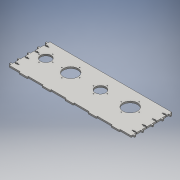
# Autodesk Inventor part: PLANO  N°1
Saved by Autodesk Inventor 2016 (Build 200138000, 138)
## iProperties
Created: 2017-09-26
Part Number: PLANO  N°1
Material: Genérico
Document SubType Name: Modeling
Designer: Alumno
Density: 1 g/cm^3
Appearance: Valor por defecto
Author: Alumno
Autodesk Inventor part; units mm, degrees
ref_plane "YZ Plane" through (0, 0, 0) normal (1, 0, 0) x (0, 1, 0)
ref_plane "XZ Plane" through (0, 0, 0) normal (0, 1, 0) x (-1, 0, 0)
ref_plane "XY Plane" through (0, 0, 0) normal (0, 0, 1) x (1, 0, 0)
sketch "Boceto1" plane through (0, 0, 0) normal (0, 0, 1) x (1, 0, 0)
  circle A0 centre (-88.2, 15) radius 27
  circle A1 centre (131.4, 15) radius 27
  circle A2 centre (21.6, 15) radius 19.5
  circle A3 centre (-180, 15) radius 19.5
  line L0 (225, 16.7667) -> (218.8, 16.7667)
  line L1 (218.8, 16.7667) -> (218.8, 15.4667)
  line L2 (218.8, 15.4667) -> (216, 15.4667)
  line L3 (216, 15.4667) -> (216, 16.7667)
  line L4 (216, 16.7667) -> (210, 16.7667)
  line L5 (210, 16.7667) -> (210, 20.1167)
  line L6 (210, 20.1167) -> (216, 20.1167)
  line L7 (216, 20.1167) -> (216, 21.4167)
  line L8 (216, 21.4167) -> (218.8, 21.4167)
  line L9 (218.8, 21.4167) -> (218.8, 20.1167)
  line L10 (218.8, 20.1167) -> (225, 20.1167)
  line L11 (225, 20.1167) -> (225, 34.3833)
  line L12 (225, 39.3833) -> (225, 53.65)
  line L13 (225, 53.65) -> (218.8, 53.65)
  line L14 (218.8, 53.65) -> (218.8, 52.35)
  line L15 (218.8, 52.35) -> (216, 52.35)
  line L16 (216, 52.35) -> (216, 53.65)
  line L17 (216, 53.65) -> (210, 53.65)
  line L18 (210, 53.65) -> (210, 57)
  line L19 (210, 57) -> (216, 57)
  line L20 (216, 57) -> (216, 58.3)
  line L21 (216, 58.3) -> (218.8, 58.3)
  line L22 (218.8, 58.3) -> (218.8, 57)
  line L23 (218.8, 57) -> (225, 57)
  line L24 (225, 57) -> (225, 63.9297)
  line L25 (225, 63.9297) -> (231, 63.9297)
  line L26 (231, 68.9297) -> (231, 63.9297)
  line L27 (225, 68.9297) -> (231, 68.9297)
  line L28 (225, 68.9297) -> (225, 75)
  line L29 (225, 75) -> (-225, 75)
  line L30 (-225, 75) -> (-225, 68.9297)
  line L31 (-225, 68.9297) -> (-231, 68.9297)
  line L32 (-231, 68.9297) -> (-231, 63.9297)
  line L33 (-231, 63.9297) -> (-225, 63.9297)
  line L34 (-225, 63.9297) -> (-225, 57)
  line L35 (-225, 57) -> (-218.8, 57)
  line L36 (-218.8, 57) -> (-218.8, 58.3)
  line L37 (-218.8, 58.3) -> (-216, 58.3)
  line L38 (-216, 58.3) -> (-216, 57)
  line L39 (-216, 57) -> (-210, 57)
  line L40 (-210, 57) -> (-210, 53.65)
  line L41 (-210, 53.65) -> (-216, 53.65)
  line L42 (-216, 53.65) -> (-216, 52.35)
  line L43 (-216, 52.35) -> (-218.8, 52.35)
  line L44 (-218.8, 52.35) -> (-218.8, 53.65)
  line L45 (-218.8, 53.65) -> (-225, 53.65)
  line L46 (-225, 53.65) -> (-225, 39.3833)
  line L47 (-225, 39.3833) -> (-231, 39.3833)
  line L48 (-231, 39.3833) -> (-231, 34.3833)
  line L49 (-231, 34.3833) -> (-225, 34.3833)
  line L50 (-225, 34.3833) -> (-225, 20.1167)
  line L51 (-225, 20.1167) -> (-218.8, 20.1167)
  line L52 (-218.8, 20.1167) -> (-218.8, 21.4167)
  line L53 (-218.8, 21.4167) -> (-216, 21.4167)
  line L54 (-216, 21.4167) -> (-216, 20.1167)
  line L55 (-216, 20.1167) -> (-210, 20.1167)
  line L56 (-210, 20.1167) -> (-210, 16.7667)
  line L57 (-210, 16.7667) -> (-216, 16.7667)
  line L58 (-216, 16.7667) -> (-216, 15.4667)
  line L59 (-216, 15.4667) -> (-218.8, 15.4667)
  line L60 (-218.8, 15.4667) -> (-218.8, 16.7667)
  line L61 (-218.8, 16.7667) -> (-225, 16.7667)
  line L62 (-225, 16.7667) -> (-225, 2.5)
  line L63 (-225, 2.5) -> (-231, 2.5)
  line L64 (-231, 2.5) -> (-231, -2.5)
  line L65 (-231, -2.5) -> (-225, -2.5)
  line L66 (-225, -2.5) -> (-225, -16.7667)
  line L67 (-225, -16.7667) -> (-218.8, -16.7667)
  line L68 (-218.8, -16.7667) -> (-218.8, -15.4667)
  line L69 (-218.8, -15.4667) -> (-216, -15.4667)
  line L70 (-216, -15.4667) -> (-216, -16.7667)
  line L71 (-216, -16.7667) -> (-210, -16.7667)
  line L72 (-210, -16.7667) -> (-210, -20.1167)
  line L73 (-210, -20.1167) -> (-216, -20.1167)
  line L74 (-216, -20.1167) -> (-216, -21.4167)
  line L75 (-216, -21.4167) -> (-218.8, -21.4167)
  line L76 (-218.8, -21.4167) -> (-218.8, -20.1167)
  line L77 (-218.8, -20.1167) -> (-225, -20.1167)
  line L78 (-225, -20.1167) -> (-225, -34.3833)
  line L79 (-225, -34.3833) -> (-231, -34.3833)
  line L80 (-231, -34.3833) -> (-231, -39.3833)
  line L81 (-231, -39.3833) -> (-225, -39.3833)
  line L82 (-225, -39.3833) -> (-225, -53.65)
  line L83 (-225, -53.65) -> (-218.8, -53.65)
  line L84 (-218.8, -53.65) -> (-218.8, -52.35)
  line L85 (-218.8, -52.35) -> (-216, -52.35)
  line L86 (-216, -52.35) -> (-216, -53.65)
  line L87 (-216, -53.65) -> (-210, -53.65)
  line L88 (-210, -53.65) -> (-210, -57)
  line L89 (-210, -57) -> (-216, -57)
  line L90 (-216, -57) -> (-216, -58.3)
  line L91 (-216, -58.3) -> (-218.8, -58.3)
  line L92 (-218.8, -58.3) -> (-218.8, -57)
  line L93 (-218.8, -57) -> (-225, -57)
  line L94 (-225, -57) -> (-225, -63.5)
  line L95 (-225, -63.5) -> (-231, -63.5)
  line L96 (-231, -63.5) -> (-231, -68.5)
  line L97 (-231, -68.5) -> (-225, -68.5)
  line L98 (-225, -68.5) -> (-225, -75)
  line L99 (-225, -75) -> (-185, -75)
  line L100 (-185, -75) -> (-185, -79)
  line L101 (-185, -79) -> (-155, -79)
  line L102 (-155, -79) -> (-155, -75)
  line L103 (-155, -75) -> (-100, -75)
  line L104 (-100, -75) -> (-100, -79)
  line L105 (-100, -79) -> (-70, -79)
  line L106 (-70, -79) -> (-70, -75)
  line L107 (-70, -75) -> (-15, -75)
  line L108 (-15, -75) -> (-15, -79)
  line L109 (-15, -79) -> (15, -79)
  line L110 (15, -79) -> (15, -75)
  line L111 (15, -75) -> (70, -75)
  line L112 (70, -75) -> (70, -79)
  line L113 (70, -79) -> (100, -79)
  line L114 (100, -79) -> (100, -75)
  line L115 (100, -75) -> (155, -75)
  line L116 (155, -79) -> (155, -75)
  line L117 (185, -79) -> (155, -79)
  line L118 (185, -75) -> (185, -79)
  line L119 (185, -75) -> (225, -75)
  line L120 (225, -75) -> (225, -68.5)
  line L121 (225, -68.5) -> (231, -68.5)
  line L122 (231, -63.5) -> (231, -68.5)
  line L123 (225, -63.5) -> (231, -63.5)
  line L124 (225, -63.5) -> (225, -57)
  line L125 (225, -57) -> (218.8, -57)
  line L126 (218.8, -57) -> (218.8, -58.3)
  line L127 (218.8, -58.3) -> (216, -58.3)
  line L128 (216, -58.3) -> (216, -57)
  line L129 (216, -57) -> (210, -57)
  line L130 (210, -57) -> (210, -53.65)
  line L131 (210, -53.65) -> (216, -53.65)
  line L132 (216, -53.65) -> (216, -52.35)
  line L133 (216, -52.35) -> (218.8, -52.35)
  line L134 (218.8, -52.35) -> (218.8, -53.65)
  line L135 (218.8, -53.65) -> (225, -53.65)
  line L136 (225, -53.65) -> (225, -39.3833)
  line L137 (225, -39.3833) -> (231, -39.3833)
  line L138 (231, -34.3833) -> (231, -39.3833)
  line L139 (225, -34.3833) -> (231, -34.3833)
  line L140 (225, -34.3833) -> (225, -20.1167)
  line L141 (225, -20.1167) -> (218.8, -20.1167)
  line L142 (218.8, -20.1167) -> (218.8, -21.4167)
  line L143 (218.8, -21.4167) -> (216, -21.4167)
  line L144 (216, -21.4167) -> (216, -20.1167)
  line L145 (216, -20.1167) -> (210, -20.1167)
  line L146 (210, -20.1167) -> (210, -16.7667)
  line L147 (210, -16.7667) -> (216, -16.7667)
  line L148 (216, -16.7667) -> (216, -15.4667)
  line L149 (216, -15.4667) -> (218.8, -15.4667)
  line L150 (218.8, -15.4667) -> (218.8, -16.7667)
  line L151 (218.8, -16.7667) -> (225, -16.7667)
  line L152 (225, -16.7667) -> (225, -2.5)
  line L153 (225, -2.5) -> (231, -2.5)
  line L154 (231, 2.5) -> (231, -2.5)
  line L155 (225, 2.5) -> (231, 2.5)
  line L156 (225, 2.5) -> (225, 16.7667)
  line L157 (225, 39.3833) -> (231, 39.3833)
  line L158 (231, 39.3833) -> (231, 34.3833)
  line L159 (231, 34.3833) -> (225, 34.3833)
  point P0 (0, 0)
  point P1 (0, 0)
  dimension "d0" = 450
  dimension "d1" = 150
  dimension "d6" = 54
  dimension "d7" = 60
  dimension "d9" = 90
  dimension "d10" = 45
  dimension "d11" = 91.8
  dimension "d12" = 39
  dimension "d14" = 90
  dimension "d15" = 39
  dimension "d16" = 90
  dimension "d17" = 14.2667
  dimension "d19" = 54
  dimension "d20" = 109.8
  dimension "d21" = 109.8
  dimension "d58" = 6.2
  dimension "d59" = 6.2
  dimension "d60" = 2.8
  dimension "d61" = 2.8
  dimension "d62" = 450
  dimension "d63" = 450
  dimension "d64" = 450
  dimension "d65" = 450
  dimension "d67" = 15
  dimension "d68" = 15
  dimension "d69" = 6
  dimension "d70" = 5
  constraints: 320 end point, 4 centre point, 2 perpendicular, 1 horizontal
  measures "d0" distance of L29.start L29.end
  measures "d1" distance between parallel lines of L103 L29
  measures "d6" diameter of A0
  measures "d7" distance from line of L29 A0.centre
  measures "d9" distance from line of L99 A3.centre
  measures "d10" distance from line of A3.centre L50
  measures "d11" distance of A0.centre A3.centre
  measures "d12" diameter of A3
  measures "d14" distance from line of L107 A2.centre
  measures "d15" diameter of A2
  measures "d16" distance from line of L115 A1.centre
  measures "d17" distance of L10.end L11.end
  measures "d19" diameter of A1
  measures "d20" distance of A2.centre A0.centre
  measures "d21" distance of A1.centre A2.centre
  measures "d58" distance of L22.end L23.end
  measures "d59" distance of L13.start L14.start
  measures "d60" distance of L15.start L16.start
  measures "d61" distance of L20.end L22.start
  measures "d62" distance from line of L120 L98.end
  measures "d63" distance between parallel lines of L30 L12
  measures "d64" distance between parallel lines of L30 L11
  measures "d65" distance between parallel lines of L30 L156
  measures "d67" distance between parallel lines of L24 L18
  measures "d68" distance between parallel lines of L11 L5
  measures "d69" distance of L12.start L157.end
  measures "d70" distance of L157.end L158.end
extrude "Extrusión1" add sketch "Boceto1" along normal blind 6
sketch "Boceto2" plane through (0, 0, 6) normal (0, 0, 1) x (1, 0, 0)
  circle A0 centre (-88.2, 15) radius 27 projected
  circle A1 centre (131.4, 15) radius 27 projected
  circle A2 centre (-180, 15) radius 19.5 projected
  circle A3 centre (21.6, 15) radius 19.5 projected
  line L0 (225, 16.7667) -> (218.8, 16.7667) projected
  line L1 (218.8, 16.7667) -> (218.8, 15.4667) projected
  line L2 (218.8, 15.4667) -> (216, 15.4667) projected
  line L3 (216, 15.4667) -> (216, 16.7667) projected
  line L4 (216, 16.7667) -> (210, 16.7667) projected
  line L5 (210, 16.7667) -> (210, 20.1167) projected
  line L6 (210, 20.1167) -> (216, 20.1167) projected
  line L7 (216, 20.1167) -> (216, 21.4167) projected
  line L8 (216, 21.4167) -> (218.8, 21.4167) projected
  line L9 (218.8, 21.4167) -> (218.8, 20.1167) projected
  line L10 (218.8, 20.1167) -> (225, 20.1167) projected
  line L11 (225, 20.1167) -> (225, 34.3833) projected
  line L12 (225, 39.3833) -> (225, 53.65) projected
  line L13 (225, 53.65) -> (218.8, 53.65) projected
  line L14 (218.8, 53.65) -> (218.8, 52.35) projected
  line L15 (218.8, 52.35) -> (216, 52.35) projected
  line L16 (216, 52.35) -> (216, 53.65) projected
  line L17 (216, 53.65) -> (210, 53.65) projected
  line L18 (210, 53.65) -> (210, 57) projected
  line L19 (210, 57) -> (216, 57) projected
  line L20 (216, 57) -> (216, 58.3) projected
  line L21 (216, 58.3) -> (218.8, 58.3) projected
  line L22 (218.8, 58.3) -> (218.8, 57) projected
  line L23 (218.8, 57) -> (225, 57) projected
  line L24 (225, 57) -> (225, 63.9297) projected
  line L25 (225, 63.9297) -> (231, 63.9297) projected
  line L26 (231, 63.9297) -> (231, 68.9297) projected
  line L27 (231, 68.9297) -> (225, 68.9297) projected
  line L28 (225, 68.9297) -> (225, 75) projected
  line L29 (225, 75) -> (-225, 75) projected
  line L30 (-225, 75) -> (-225, 68.9297) projected
  line L31 (-225, 68.9297) -> (-231, 68.9297) projected
  line L32 (-231, 68.9297) -> (-231, 63.9297) projected
  line L33 (-231, 63.9297) -> (-225, 63.9297) projected
  line L34 (-225, 63.9297) -> (-225, 57) projected
  line L35 (-225, 57) -> (-218.8, 57) projected
  line L36 (-218.8, 57) -> (-218.8, 58.3) projected
  line L37 (-218.8, 58.3) -> (-216, 58.3) projected
  line L38 (-216, 58.3) -> (-216, 57) projected
  line L39 (-216, 57) -> (-210, 57) projected
  line L40 (-210, 57) -> (-210, 53.65) projected
  line L41 (-210, 53.65) -> (-216, 53.65) projected
  line L42 (-216, 53.65) -> (-216, 52.35) projected
  line L43 (-216, 52.35) -> (-218.8, 52.35) projected
  line L44 (-218.8, 52.35) -> (-218.8, 53.65) projected
  line L45 (-218.8, 53.65) -> (-225, 53.65) projected
  line L46 (-225, 53.65) -> (-225, 39.3833) projected
  line L47 (-225, 39.3833) -> (-231, 39.3833) projected
  line L48 (-231, 39.3833) -> (-231, 34.3833) projected
  line L49 (-231, 34.3833) -> (-225, 34.3833) projected
  line L50 (-225, 34.3833) -> (-225, 20.1167) projected
  line L51 (-225, 20.1167) -> (-218.8, 20.1167) projected
  line L52 (-218.8, 20.1167) -> (-218.8, 21.4167) projected
  line L53 (-218.8, 21.4167) -> (-216, 21.4167) projected
  line L54 (-216, 21.4167) -> (-216, 20.1167) projected
  line L55 (-216, 20.1167) -> (-210, 20.1167) projected
  line L56 (-210, 20.1167) -> (-210, 16.7667) projected
  line L57 (-210, 16.7667) -> (-216, 16.7667) projected
  line L58 (-216, 16.7667) -> (-216, 15.4667) projected
  line L59 (-216, 15.4667) -> (-218.8, 15.4667) projected
  line L60 (-218.8, 15.4667) -> (-218.8, 16.7667) projected
  line L61 (-218.8, 16.7667) -> (-225, 16.7667) projected
  line L62 (-225, 16.7667) -> (-225, 2.5) projected
  line L63 (-225, 2.5) -> (-231, 2.5) projected
  line L64 (-231, 2.5) -> (-231, -2.5) projected
  line L65 (-231, -2.5) -> (-225, -2.5) projected
  line L66 (-225, -2.5) -> (-225, -16.7667) projected
  line L67 (-225, -16.7667) -> (-218.8, -16.7667) projected
  line L68 (-218.8, -16.7667) -> (-218.8, -15.4667) projected
  line L69 (-218.8, -15.4667) -> (-216, -15.4667) projected
  line L70 (-216, -15.4667) -> (-216, -16.7667) projected
  line L71 (-216, -16.7667) -> (-210, -16.7667) projected
  line L72 (-210, -16.7667) -> (-210, -20.1167) projected
  line L73 (-210, -20.1167) -> (-216, -20.1167) projected
  line L74 (-216, -20.1167) -> (-216, -21.4167) projected
  line L75 (-216, -21.4167) -> (-218.8, -21.4167) projected
  line L76 (-218.8, -21.4167) -> (-218.8, -20.1167) projected
  line L77 (-218.8, -20.1167) -> (-225, -20.1167) projected
  line L78 (-225, -20.1167) -> (-225, -34.3833) projected
  line L79 (-225, -34.3833) -> (-231, -34.3833) projected
  line L80 (-231, -34.3833) -> (-231, -39.3833) projected
  line L81 (-231, -39.3833) -> (-225, -39.3833) projected
  line L82 (-225, -39.3833) -> (-225, -53.65) projected
  line L83 (-225, -53.65) -> (-218.8, -53.65) projected
  line L84 (-218.8, -53.65) -> (-218.8, -52.35) projected
  line L85 (-218.8, -52.35) -> (-216, -52.35) projected
  line L86 (-216, -52.35) -> (-216, -53.65) projected
  line L87 (-216, -53.65) -> (-210, -53.65) projected
  line L88 (-210, -53.65) -> (-210, -57) projected
  line L89 (-210, -57) -> (-216, -57) projected
  line L90 (-216, -57) -> (-216, -58.3) projected
  line L91 (-216, -58.3) -> (-218.8, -58.3) projected
  line L92 (-218.8, -58.3) -> (-218.8, -57) projected
  line L93 (-218.8, -57) -> (-225, -57) projected
  line L94 (-225, -57) -> (-225, -63.5) projected
  line L95 (-225, -63.5) -> (-231, -63.5) projected
  line L96 (-231, -63.5) -> (-231, -68.5) projected
  line L97 (-231, -68.5) -> (-225, -68.5) projected
  line L98 (-225, -68.5) -> (-225, -75) projected
  line L99 (-225, -75) -> (-185, -75) projected
  line L100 (-185, -75) -> (-185, -79) projected
  line L101 (-185, -79) -> (-155, -79) projected
  line L102 (-155, -79) -> (-155, -75) projected
  line L103 (-155, -75) -> (-100, -75) projected
  line L104 (-100, -75) -> (-100, -79) projected
  line L105 (-100, -79) -> (-70, -79) projected
  line L106 (-70, -79) -> (-70, -75) projected
  line L107 (-70, -75) -> (-15, -75) projected
  line L108 (-15, -75) -> (-15, -79) projected
  line L109 (-15, -79) -> (15, -79) projected
  line L110 (15, -79) -> (15, -75) projected
  line L111 (15, -75) -> (70, -75) projected
  line L112 (70, -75) -> (70, -79) projected
  line L113 (70, -79) -> (100, -79) projected
  line L114 (100, -79) -> (100, -75) projected
  line L115 (100, -75) -> (155, -75) projected
  line L116 (155, -75) -> (155, -79) projected
  line L117 (155, -79) -> (185, -79) projected
  line L118 (185, -79) -> (185, -75) projected
  line L119 (185, -75) -> (225, -75) projected
  line L120 (225, -75) -> (225, -68.5) projected
  line L121 (225, -68.5) -> (231, -68.5) projected
  line L122 (231, -68.5) -> (231, -63.5) projected
  line L123 (231, -63.5) -> (225, -63.5) projected
  line L124 (225, -63.5) -> (225, -57) projected
  line L125 (225, -57) -> (218.8, -57) projected
  line L126 (218.8, -57) -> (218.8, -58.3) projected
  line L127 (218.8, -58.3) -> (216, -58.3) projected
  line L128 (216, -58.3) -> (216, -57) projected
  line L129 (216, -57) -> (210, -57) projected
  line L130 (210, -57) -> (210, -53.65) projected
  line L131 (210, -53.65) -> (216, -53.65) projected
  line L132 (216, -53.65) -> (216, -52.35) projected
  line L133 (216, -52.35) -> (218.8, -52.35) projected
  line L134 (218.8, -52.35) -> (218.8, -53.65) projected
  line L135 (218.8, -53.65) -> (225, -53.65) projected
  line L136 (225, -53.65) -> (225, -39.3833) projected
  line L137 (225, -39.3833) -> (231, -39.3833) projected
  line L138 (231, -39.3833) -> (231, -34.3833) projected
  line L139 (231, -34.3833) -> (225, -34.3833) projected
  line L140 (225, -34.3833) -> (225, -20.1167) projected
  line L141 (225, -20.1167) -> (218.8, -20.1167) projected
  line L142 (218.8, -20.1167) -> (218.8, -21.4167) projected
  line L143 (218.8, -21.4167) -> (216, -21.4167) projected
  line L144 (216, -21.4167) -> (216, -20.1167) projected
  line L145 (216, -20.1167) -> (210, -20.1167) projected
  line L146 (210, -20.1167) -> (210, -16.7667) projected
  line L147 (210, -16.7667) -> (216, -16.7667) projected
  line L148 (216, -16.7667) -> (216, -15.4667) projected
  line L149 (216, -15.4667) -> (218.8, -15.4667) projected
  line L150 (218.8, -15.4667) -> (218.8, -16.7667) projected
  line L151 (218.8, -16.7667) -> (225, -16.7667) projected
  line L152 (225, -16.7667) -> (225, -2.5) projected
  line L153 (225, -2.5) -> (231, -2.5) projected
  line L154 (231, -2.5) -> (231, 2.5) projected
  line L155 (231, 2.5) -> (225, 2.5) projected
  line L156 (225, 2.5) -> (225, 16.7667) projected
  circle A4 centre (-88.2, 48) radius 1.5
  circle A5 centre (-121.2, 15) radius 1.5
  circle A6 centre (-88.2, -18) radius 1.5
  circle A7 centre (-55.2, 15) radius 1.5
  circle A8 centre (131.4, 48) radius 1.5
  circle A9 centre (98.4, 15) radius 1.5
  circle A10 centre (131.4, -18) radius 1.5
  circle A11 centre (164.4, 15) radius 1.5
  line L157 (225, 34.3833) -> (231, 34.3833) projected
  line L158 (231, 34.3833) -> (231, 39.3833) projected
  line L159 (231, 39.3833) -> (225, 39.3833) projected
  point P0 (0, 0)
  dimension "d25" = 3
  dimension "d26" = 33
  dimension "d29" = 360
  dimension "d31" = 3
  dimension "d32" = 33
  dimension "d35" = 360
  constraints: 8 centre point, 18 other
  measures "d25" diameter of A4
  measures "d26" distance of A0.centre A4.centre
  measures "d31" diameter of A8
  measures "d32" distance of A1.centre A8.centre
extrude "Extrusión2" cut sketch "Boceto2" against normal blind 6 contours A4 | A5 | A6 | A7 | A8 | A9 | A10 | A11
sketch "Boceto3" plane through (0, 0, 6) normal (0, 0, 1) x (1, 0, 0)
  circle A0 centre (131.4, -18) radius 1.5 projected
  circle A1 centre (131.4, 48) radius 1.5 projected
  circle A2 centre (-88.2, -18) radius 1.5 projected
  circle A3 centre (-88.2, 48) radius 1.5 projected
  circle A4 centre (-121.2, 15) radius 1.5 projected
  circle A5 centre (-55.2, 15) radius 1.5 projected
  circle A6 centre (98.4, 15) radius 1.5 projected
  circle A7 centre (164.4, 15) radius 1.5 projected
  circle A8 centre (-88.2, 15) radius 27 projected
  circle A9 centre (131.4, 15) radius 27 projected
  circle A10 centre (-180, 15) radius 19.5 projected
  circle A11 centre (21.6, 15) radius 19.5 projected
  line L0 (225, 16.7667) -> (218.8, 16.7667) projected
  line L1 (218.8, 16.7667) -> (218.8, 15.4667) projected
  line L2 (218.8, 15.4667) -> (216, 15.4667) projected
  line L3 (216, 15.4667) -> (216, 16.7667) projected
  line L4 (216, 16.7667) -> (210, 16.7667) projected
  line L5 (210, 16.7667) -> (210, 20.1167) projected
  line L6 (210, 20.1167) -> (216, 20.1167) projected
  line L7 (216, 20.1167) -> (216, 21.4167) projected
  line L8 (216, 21.4167) -> (218.8, 21.4167) projected
  line L9 (218.8, 21.4167) -> (218.8, 20.1167) projected
  line L10 (218.8, 20.1167) -> (225, 20.1167) projected
  line L11 (225, 20.1167) -> (225, 34.3833) projected
  line L12 (225, 39.3833) -> (225, 53.65) projected
  line L13 (225, 53.65) -> (218.8, 53.65) projected
  line L14 (218.8, 53.65) -> (218.8, 52.35) projected
  line L15 (218.8, 52.35) -> (216, 52.35) projected
  line L16 (216, 52.35) -> (216, 53.65) projected
  line L17 (216, 53.65) -> (210, 53.65) projected
  line L18 (210, 53.65) -> (210, 57) projected
  line L19 (210, 57) -> (216, 57) projected
  line L20 (216, 57) -> (216, 58.3) projected
  line L21 (216, 58.3) -> (218.8, 58.3) projected
  line L22 (218.8, 58.3) -> (218.8, 57) projected
  line L23 (218.8, 57) -> (225, 57) projected
  line L24 (225, 57) -> (225, 63.9297) projected
  line L25 (225, 63.9297) -> (231, 63.9297) projected
  line L26 (231, 63.9297) -> (231, 68.9297) projected
  line L27 (231, 68.9297) -> (225, 68.9297) projected
  line L28 (225, 68.9297) -> (225, 75) projected
  line L29 (225, 75) -> (-225, 75) projected
  line L30 (-225, 75) -> (-225, 68.9297) projected
  line L31 (-225, 68.9297) -> (-231, 68.9297) projected
  line L32 (-231, 68.9297) -> (-231, 63.9297) projected
  line L33 (-231, 63.9297) -> (-225, 63.9297) projected
  line L34 (-225, 63.9297) -> (-225, 57) projected
  line L35 (-225, 57) -> (-218.8, 57) projected
  line L36 (-218.8, 57) -> (-218.8, 58.3) projected
  line L37 (-218.8, 58.3) -> (-216, 58.3) projected
  line L38 (-216, 58.3) -> (-216, 57) projected
  line L39 (-216, 57) -> (-210, 57) projected
  line L40 (-210, 57) -> (-210, 53.65) projected
  line L41 (-210, 53.65) -> (-216, 53.65) projected
  line L42 (-216, 53.65) -> (-216, 52.35) projected
  line L43 (-216, 52.35) -> (-218.8, 52.35) projected
  line L44 (-218.8, 52.35) -> (-218.8, 53.65) projected
  line L45 (-218.8, 53.65) -> (-225, 53.65) projected
  line L46 (-225, 53.65) -> (-225, 39.3833) projected
  line L47 (-225, 39.3833) -> (-231, 39.3833) projected
  line L48 (-231, 39.3833) -> (-231, 34.3833) projected
  line L49 (-231, 34.3833) -> (-225, 34.3833) projected
  line L50 (-225, 34.3833) -> (-225, 20.1167) projected
  line L51 (-225, 20.1167) -> (-218.8, 20.1167) projected
  line L52 (-218.8, 20.1167) -> (-218.8, 21.4167) projected
  line L53 (-218.8, 21.4167) -> (-216, 21.4167) projected
  line L54 (-216, 21.4167) -> (-216, 20.1167) projected
  line L55 (-216, 20.1167) -> (-210, 20.1167) projected
  line L56 (-210, 20.1167) -> (-210, 16.7667) projected
  line L57 (-210, 16.7667) -> (-216, 16.7667) projected
  line L58 (-216, 16.7667) -> (-216, 15.4667) projected
  line L59 (-216, 15.4667) -> (-218.8, 15.4667) projected
  line L60 (-218.8, 15.4667) -> (-218.8, 16.7667) projected
  line L61 (-218.8, 16.7667) -> (-225, 16.7667) projected
  line L62 (-225, 16.7667) -> (-225, 2.5) projected
  line L63 (-225, 2.5) -> (-231, 2.5) projected
  line L64 (-231, 2.5) -> (-231, -2.5) projected
  line L65 (-231, -2.5) -> (-225, -2.5) projected
  line L66 (-225, -2.5) -> (-225, -16.7667) projected
  line L67 (-225, -16.7667) -> (-218.8, -16.7667) projected
  line L68 (-218.8, -16.7667) -> (-218.8, -15.4667) projected
  line L69 (-218.8, -15.4667) -> (-216, -15.4667) projected
  line L70 (-216, -15.4667) -> (-216, -16.7667) projected
  line L71 (-216, -16.7667) -> (-210, -16.7667) projected
  line L72 (-210, -16.7667) -> (-210, -20.1167) projected
  line L73 (-210, -20.1167) -> (-216, -20.1167) projected
  line L74 (-216, -20.1167) -> (-216, -21.4167) projected
  line L75 (-216, -21.4167) -> (-218.8, -21.4167) projected
  line L76 (-218.8, -21.4167) -> (-218.8, -20.1167) projected
  line L77 (-218.8, -20.1167) -> (-225, -20.1167) projected
  line L78 (-225, -20.1167) -> (-225, -34.3833) projected
  line L79 (-225, -34.3833) -> (-231, -34.3833) projected
  line L80 (-231, -34.3833) -> (-231, -39.3833) projected
  line L81 (-231, -39.3833) -> (-225, -39.3833) projected
  line L82 (-225, -39.3833) -> (-225, -53.65) projected
  line L83 (-225, -53.65) -> (-218.8, -53.65) projected
  line L84 (-218.8, -53.65) -> (-218.8, -52.35) projected
  line L85 (-218.8, -52.35) -> (-216, -52.35) projected
  line L86 (-216, -52.35) -> (-216, -53.65) projected
  line L87 (-216, -53.65) -> (-210, -53.65) projected
  line L88 (-210, -53.65) -> (-210, -57) projected
  line L89 (-210, -57) -> (-216, -57) projected
  line L90 (-216, -57) -> (-216, -58.3) projected
  line L91 (-216, -58.3) -> (-218.8, -58.3) projected
  line L92 (-218.8, -58.3) -> (-218.8, -57) projected
  line L93 (-218.8, -57) -> (-225, -57) projected
  line L94 (-225, -57) -> (-225, -63.5) projected
  line L95 (-225, -63.5) -> (-231, -63.5) projected
  line L96 (-231, -63.5) -> (-231, -68.5) projected
  line L97 (-231, -68.5) -> (-225, -68.5) projected
  line L98 (-225, -68.5) -> (-225, -75) projected
  line L99 (-225, -75) -> (-185, -75) projected
  line L100 (-185, -75) -> (-185, -79) projected
  line L101 (-185, -79) -> (-155, -79) projected
  line L102 (-155, -79) -> (-155, -75) projected
  line L103 (-155, -75) -> (-100, -75) projected
  line L104 (-100, -75) -> (-100, -79) projected
  line L105 (-100, -79) -> (-70, -79) projected
  line L106 (-70, -79) -> (-70, -75) projected
  line L107 (-70, -75) -> (-15, -75) projected
  line L108 (-15, -75) -> (-15, -79) projected
  line L109 (-15, -79) -> (15, -79) projected
  line L110 (15, -79) -> (15, -75) projected
  line L111 (15, -75) -> (70, -75) projected
  line L112 (70, -75) -> (70, -79) projected
  line L113 (70, -79) -> (100, -79) projected
  line L114 (100, -79) -> (100, -75) projected
  line L115 (100, -75) -> (155, -75) projected
  line L116 (155, -75) -> (155, -79) projected
  line L117 (155, -79) -> (185, -79) projected
  line L118 (185, -79) -> (185, -75) projected
  line L119 (185, -75) -> (225, -75) projected
  line L120 (225, -75) -> (225, -68.5) projected
  line L121 (225, -68.5) -> (231, -68.5) projected
  line L122 (231, -68.5) -> (231, -63.5) projected
  line L123 (231, -63.5) -> (225, -63.5) projected
  line L124 (225, -63.5) -> (225, -57) projected
  line L125 (225, -57) -> (218.8, -57) projected
  line L126 (218.8, -57) -> (218.8, -58.3) projected
  line L127 (218.8, -58.3) -> (216, -58.3) projected
  line L128 (216, -58.3) -> (216, -57) projected
  line L129 (216, -57) -> (210, -57) projected
  line L130 (210, -57) -> (210, -53.65) projected
  line L131 (210, -53.65) -> (216, -53.65) projected
  line L132 (216, -53.65) -> (216, -52.35) projected
  line L133 (216, -52.35) -> (218.8, -52.35) projected
  line L134 (218.8, -52.35) -> (218.8, -53.65) projected
  line L135 (218.8, -53.65) -> (225, -53.65) projected
  line L136 (225, -53.65) -> (225, -39.3833) projected
  line L137 (225, -39.3833) -> (231, -39.3833) projected
  line L138 (231, -39.3833) -> (231, -34.3833) projected
  line L139 (231, -34.3833) -> (225, -34.3833) projected
  line L140 (225, -34.3833) -> (225, -20.1167) projected
  line L141 (225, -20.1167) -> (218.8, -20.1167) projected
  line L142 (218.8, -20.1167) -> (218.8, -21.4167) projected
  line L143 (218.8, -21.4167) -> (216, -21.4167) projected
  line L144 (216, -21.4167) -> (216, -20.1167) projected
  line L145 (216, -20.1167) -> (210, -20.1167) projected
  line L146 (210, -20.1167) -> (210, -16.7667) projected
  line L147 (210, -16.7667) -> (216, -16.7667) projected
  line L148 (216, -16.7667) -> (216, -15.4667) projected
  line L149 (216, -15.4667) -> (218.8, -15.4667) projected
  line L150 (218.8, -15.4667) -> (218.8, -16.7667) projected
  line L151 (218.8, -16.7667) -> (225, -16.7667) projected
  line L152 (225, -16.7667) -> (225, -2.5) projected
  line L153 (225, -2.5) -> (231, -2.5) projected
  line L154 (231, -2.5) -> (231, 2.5) projected
  line L155 (231, 2.5) -> (225, 2.5) projected
  line L156 (225, 2.5) -> (225, 16.7667) projected
  circle A12 centre (-180, 40.5) radius 1.5
  circle A13 centre (-205.5, 15) radius 1.5
  circle A14 centre (-180, -10.5) radius 1.5
  circle A15 centre (-154.5, 15) radius 1.5
  circle A16 centre (21.6, 40.5) radius 1.5
  circle A17 centre (-3.9, 15) radius 1.5
  circle A18 centre (21.6, -10.5) radius 1.5
  circle A19 centre (47.1, 15) radius 1.5
  line L157 (225, 34.3833) -> (231, 34.3833) projected
  line L158 (231, 34.3833) -> (231, 39.3833) projected
  line L159 (231, 39.3833) -> (225, 39.3833) projected
  point P0 (0, 0)
  dimension "d44" = 3
  dimension "d45" = 25.5
  dimension "d48" = 360
  dimension "d50" = 3
  dimension "d51" = 25.5
  dimension "d54" = 360
  constraints: 8 centre point, 18 other
  measures "d44" diameter of A12
  measures "d45" distance of A10.centre A12.centre
  measures "d50" diameter of A16
  measures "d51" distance of A11.centre A16.centre
extrude "Extrusión3" cut sketch "Boceto3" against normal blind 6 contours A12 | A13 | A14 | A15 | A16 | A17 | A18 | A19
sketch "Boceto6" plane through (0, 0, 6) normal (0, 0, 1) x (1, 0, 0)
  circle A0 centre (21.6, -10.5) radius 1.5 projected
  circle A1 centre (21.6, 40.5) radius 1.5 projected
  circle A2 centre (-180, -10.5) radius 1.5 projected
  circle A3 centre (-180, 40.5) radius 1.5 projected
  circle A4 centre (-205.5, 15) radius 1.5 projected
  circle A5 centre (-154.5, 15) radius 1.5 projected
  circle A6 centre (-3.9, 15) radius 1.5 projected
  circle A7 centre (47.1, 15) radius 1.5 projected
  circle A8 centre (131.4, -18) radius 1.5 projected
  circle A9 centre (131.4, 48) radius 1.5 projected
  circle A10 centre (-88.2, -18) radius 1.5 projected
  circle A11 centre (-88.2, 48) radius 1.5 projected
  circle A12 centre (-121.2, 15) radius 1.5 projected
  circle A13 centre (-55.2, 15) radius 1.5 projected
  circle A14 centre (98.4, 15) radius 1.5 projected
  circle A15 centre (164.4, 15) radius 1.5 projected
  circle A16 centre (-88.2, 15) radius 27 projected
  circle A17 centre (131.4, 15) radius 27 projected
  circle A18 centre (-180, 15) radius 19.5 projected
  circle A19 centre (21.6, 15) radius 19.5 projected
  line L0 (225, 16.7667) -> (218.8, 16.7667) projected
  line L1 (218.8, 16.7667) -> (218.8, 15.4667) projected
  line L2 (218.8, 15.4667) -> (216, 15.4667) projected
  line L3 (216, 15.4667) -> (216, 16.7667) projected
  line L4 (216, 16.7667) -> (210, 16.7667) projected
  line L5 (210, 16.7667) -> (210, 20.1167) projected
  line L6 (210, 20.1167) -> (216, 20.1167) projected
  line L7 (216, 20.1167) -> (216, 21.4167) projected
  line L8 (216, 21.4167) -> (218.8, 21.4167) projected
  line L9 (218.8, 21.4167) -> (218.8, 20.1167) projected
  line L10 (218.8, 20.1167) -> (225, 20.1167) projected
  line L11 (225, 20.1167) -> (225, 34.3833) projected
  line L12 (225, 39.3833) -> (225, 53.65) projected
  line L13 (225, 53.65) -> (218.8, 53.65) projected
  line L14 (218.8, 53.65) -> (218.8, 52.35) projected
  line L15 (218.8, 52.35) -> (216, 52.35) projected
  line L16 (216, 52.35) -> (216, 53.65) projected
  line L17 (216, 53.65) -> (210, 53.65) projected
  line L18 (210, 53.65) -> (210, 57) projected
  line L19 (210, 57) -> (216, 57) projected
  line L20 (216, 57) -> (216, 58.3) projected
  line L21 (216, 58.3) -> (218.8, 58.3) projected
  line L22 (218.8, 58.3) -> (218.8, 57) projected
  line L23 (218.8, 57) -> (225, 57) projected
  line L24 (225, 57) -> (225, 63.9297) projected
  line L25 (225, 63.9297) -> (231, 63.9297) projected
  line L26 (231, 63.9297) -> (231, 68.9297) projected
  line L27 (231, 68.9297) -> (225, 68.9297) projected
  line L28 (225, 68.9297) -> (225, 75) projected
  line L29 (225, 75) -> (-225, 75) projected
  line L30 (-225, 75) -> (-225, 68.9297) projected
  line L31 (-225, 68.9297) -> (-231, 68.9297) projected
  line L32 (-231, 68.9297) -> (-231, 63.9297) projected
  line L33 (-231, 63.9297) -> (-225, 63.9297) projected
  line L34 (-225, 63.9297) -> (-225, 57) projected
  line L35 (-225, 57) -> (-218.8, 57) projected
  line L36 (-218.8, 57) -> (-218.8, 58.3) projected
  line L37 (-218.8, 58.3) -> (-216, 58.3) projected
  line L38 (-216, 58.3) -> (-216, 57) projected
  line L39 (-216, 57) -> (-210, 57) projected
  line L40 (-210, 57) -> (-210, 53.65) projected
  line L41 (-210, 53.65) -> (-216, 53.65) projected
  line L42 (-216, 53.65) -> (-216, 52.35) projected
  line L43 (-216, 52.35) -> (-218.8, 52.35) projected
  line L44 (-218.8, 52.35) -> (-218.8, 53.65) projected
  line L45 (-218.8, 53.65) -> (-225, 53.65) projected
  line L46 (-225, 53.65) -> (-225, 39.3833) projected
  line L47 (-225, 39.3833) -> (-231, 39.3833) projected
  line L48 (-231, 39.3833) -> (-231, 34.3833) projected
  line L49 (-231, 34.3833) -> (-225, 34.3833) projected
  line L50 (-225, 34.3833) -> (-225, 20.1167) projected
  line L51 (-225, 20.1167) -> (-218.8, 20.1167) projected
  line L52 (-218.8, 20.1167) -> (-218.8, 21.4167) projected
  line L53 (-218.8, 21.4167) -> (-216, 21.4167) projected
  line L54 (-216, 21.4167) -> (-216, 20.1167) projected
  line L55 (-216, 20.1167) -> (-210, 20.1167) projected
  line L56 (-210, 20.1167) -> (-210, 16.7667) projected
  line L57 (-210, 16.7667) -> (-216, 16.7667) projected
  line L58 (-216, 16.7667) -> (-216, 15.4667) projected
  line L59 (-216, 15.4667) -> (-218.8, 15.4667) projected
  line L60 (-218.8, 15.4667) -> (-218.8, 16.7667) projected
  line L61 (-218.8, 16.7667) -> (-225, 16.7667) projected
  line L62 (-225, 16.7667) -> (-225, 2.5) projected
  line L63 (-225, 2.5) -> (-231, 2.5) projected
  line L64 (-231, 2.5) -> (-231, -2.5) projected
  line L65 (-231, -2.5) -> (-225, -2.5) projected
  line L66 (-225, -2.5) -> (-225, -16.7667) projected
  line L67 (-225, -16.7667) -> (-218.8, -16.7667) projected
  line L68 (-218.8, -16.7667) -> (-218.8, -15.4667) projected
  line L69 (-218.8, -15.4667) -> (-216, -15.4667) projected
  line L70 (-216, -15.4667) -> (-216, -16.7667) projected
  line L71 (-216, -16.7667) -> (-210, -16.7667) projected
  line L72 (-210, -16.7667) -> (-210, -20.1167) projected
  line L73 (-210, -20.1167) -> (-216, -20.1167) projected
  line L74 (-216, -20.1167) -> (-216, -21.4167) projected
  line L75 (-216, -21.4167) -> (-218.8, -21.4167) projected
  line L76 (-218.8, -21.4167) -> (-218.8, -20.1167) projected
  line L77 (-218.8, -20.1167) -> (-225, -20.1167) projected
  line L78 (-225, -20.1167) -> (-225, -34.3833) projected
  line L79 (-225, -34.3833) -> (-231, -34.3833) projected
  line L80 (-231, -34.3833) -> (-231, -39.3833) projected
  line L81 (-231, -39.3833) -> (-225, -39.3833) projected
  line L82 (-225, -39.3833) -> (-225, -53.65) projected
  line L83 (-225, -53.65) -> (-218.8, -53.65) projected
  line L84 (-218.8, -53.65) -> (-218.8, -52.35) projected
  line L85 (-218.8, -52.35) -> (-216, -52.35) projected
  line L86 (-216, -52.35) -> (-216, -53.65) projected
  line L87 (-216, -53.65) -> (-210, -53.65) projected
  line L88 (-210, -53.65) -> (-210, -57) projected
  line L89 (-210, -57) -> (-216, -57) projected
  line L90 (-216, -57) -> (-216, -58.3) projected
  line L91 (-216, -58.3) -> (-218.8, -58.3) projected
  line L92 (-218.8, -58.3) -> (-218.8, -57) projected
  line L93 (-218.8, -57) -> (-225, -57) projected
  line L94 (-225, -57) -> (-225, -63.5) projected
  line L95 (-225, -63.5) -> (-231, -63.5) projected
  line L96 (-231, -63.5) -> (-231, -68.5) projected
  line L97 (-231, -68.5) -> (-225, -68.5) projected
  line L98 (-225, -68.5) -> (-225, -75) projected
  line L99 (-225, -75) -> (-185, -75) projected
  line L100 (-185, -75) -> (-185, -79) projected
  line L101 (-185, -79) -> (-155, -79) projected
  line L102 (-155, -79) -> (-155, -75) projected
  line L103 (-155, -75) -> (-100, -75) projected
  line L104 (-100, -75) -> (-100, -79) projected
  line L105 (-100, -79) -> (-70, -79) projected
  line L106 (-70, -79) -> (-70, -75) projected
  line L107 (-70, -75) -> (-15, -75) projected
  line L108 (-15, -75) -> (-15, -79) projected
  line L109 (-15, -79) -> (15, -79) projected
  line L110 (15, -79) -> (15, -75) projected
  line L111 (15, -75) -> (70, -75) projected
  line L112 (70, -75) -> (70, -79) projected
  line L113 (70, -79) -> (100, -79) projected
  line L114 (100, -79) -> (100, -75) projected
  line L115 (100, -75) -> (155, -75) projected
  line L116 (155, -75) -> (155, -79) projected
  line L117 (155, -79) -> (185, -79) projected
  line L118 (185, -79) -> (185, -75) projected
  line L119 (185, -75) -> (225, -75) projected
  line L120 (225, -75) -> (225, -68.5) projected
  line L121 (225, -68.5) -> (231, -68.5) projected
  line L122 (231, -68.5) -> (231, -63.5) projected
  line L123 (231, -63.5) -> (225, -63.5) projected
  line L124 (225, -63.5) -> (225, -57) projected
  line L125 (225, -57) -> (218.8, -57) projected
  line L126 (218.8, -57) -> (218.8, -58.3) projected
  line L127 (218.8, -58.3) -> (216, -58.3) projected
  line L128 (216, -58.3) -> (216, -57) projected
  line L129 (216, -57) -> (210, -57) projected
  line L130 (210, -57) -> (210, -53.65) projected
  line L131 (210, -53.65) -> (216, -53.65) projected
  line L132 (216, -53.65) -> (216, -52.35) projected
  line L133 (216, -52.35) -> (218.8, -52.35) projected
  line L134 (218.8, -52.35) -> (218.8, -53.65) projected
  line L135 (218.8, -53.65) -> (225, -53.65) projected
  line L136 (225, -53.65) -> (225, -39.3833) projected
  line L137 (225, -39.3833) -> (231, -39.3833) projected
  line L138 (231, -39.3833) -> (231, -34.3833) projected
  line L139 (231, -34.3833) -> (225, -34.3833) projected
  line L140 (225, -34.3833) -> (225, -20.1167) projected
  line L141 (225, -20.1167) -> (218.8, -20.1167) projected
  line L142 (218.8, -20.1167) -> (218.8, -21.4167) projected
  line L143 (218.8, -21.4167) -> (216, -21.4167) projected
  line L144 (216, -21.4167) -> (216, -20.1167) projected
  line L145 (216, -20.1167) -> (210, -20.1167) projected
  line L146 (210, -20.1167) -> (210, -16.7667) projected
  line L147 (210, -16.7667) -> (216, -16.7667) projected
  line L148 (216, -16.7667) -> (216, -15.4667) projected
  line L149 (216, -15.4667) -> (218.8, -15.4667) projected
  line L150 (218.8, -15.4667) -> (218.8, -16.7667) projected
  line L151 (218.8, -16.7667) -> (225, -16.7667) projected
  line L152 (225, -16.7667) -> (225, -2.5) projected
  line L153 (225, -2.5) -> (231, -2.5) projected
  line L154 (231, -2.5) -> (231, 2.5) projected
  line L155 (231, 2.5) -> (225, 2.5) projected
  line L156 (225, 2.5) -> (225, 16.7667) projected
  line L157 (225, -75) -> (225, 78.5131)
  line L158 (210, -57) -> (210, 91.546)
  line L159 (225, 34.3833) -> (231, 34.3833) projected
  line L160 (231, 34.3833) -> (231, 39.3833) projected
  line L161 (231, 39.3833) -> (225, 39.3833) projected
  point P0 (0, 0)
  constraints: 4 end point, 2 vertical
